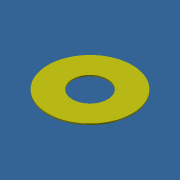
# Autodesk Inventor part: plancha
Saved by Autodesk Inventor 2014 (Build 180170000, 170)
## iProperties
Created: 2014-03-15
Part Number: plancha
Material: Generic
Document SubType Name: Modeling
Designer: Lefo
Density: 1 g/cm^3
Appearance: Default
Author: Lefo
Autodesk Inventor part; units mm, degrees
ref_plane "YZ Plane" through (0, 0, 0) normal (1, 0, 0) x (0, 1, 0)
ref_plane "XZ Plane" through (0, 0, 0) normal (0, 1, 0) x (-1, 0, 0)
ref_plane "XY Plane" through (0, 0, 0) normal (0, 0, 1) x (1, 0, 0)
sketch "Sketch1" plane through (0, 0, 0) normal (0, 1, 0) x (-1, 0, 0)
  line L0 (1200, -600) -> (-1200, -600)
  line L1 (-1200, -600) -> (-1200, 600)
  line L2 (-1200, 600) -> (1200, 600)
  line L3 (1200, 600) -> (1200, -600)
  line L4 (1200, -600) -> (-1200, 600) construction
  line L5 (-1200, -600) -> (1200, 600) construction
  circle A0 centre (0, 0) radius 130 construction
  circle A1 centre (0, 0) radius 325 construction
  line L6 (0, 325) -> (309.0934, 100.4305) construction
  line L7 (309.0934, 100.4305) -> (191.0302, -262.9305) construction
  line L8 (191.0302, -262.9305) -> (-191.0302, -262.9305) construction
  line L9 (-191.0302, -262.9305) -> (-309.0934, 100.4305) construction
  line L10 (-309.0934, 100.4305) -> (0, 325) construction
  line L11 (0, 0) -> (0, 325) construction
  line L12 (0, 0) -> (-309.0934, 100.4305) construction
  line L13 (0, 0) -> (-191.0302, -262.9305) construction
  line L14 (0, 0) -> (309.0934, 100.4305) construction
  line L15 (0, 0) -> (191.0302, -262.9305) construction
  arc A2 (-15.7737, 293.9464) -> (0, 0) centre (281.4583, 162.5) ccw
  arc A3 (224.7845, 110.9324) -> (0, 0) centre (230.7976, -184.461) ccw
  arc A4 (275.3692, 201.188) -> (35.5667, 329.5753) centre (50.8772, 70.0265) ccw
  arc A5 (224.7845, 110.9324) -> (275.3692, 201.188) centre (223.5633, 170.92) ccw
  arc A6 (35.5667, 329.5753) -> (-15.7737, 293.9464) centre (39.0999, 269.6794) ccw
  arc A7 (-284.434, 75.8328) -> (0, 0) centre (-67.5713, 317.898) ccw
  arc A8 (-36.0407, 248.0627) -> (0, 0) centre (246.7532, 162.5) ccw
  arc A9 (-106.2474, 324.0622) -> (-302.454, 135.6703) centre (-50.8772, 70.0265) ccw
  arc A10 (-36.0407, 248.0627) -> (-106.2474, 324.0622) centre (-93.4697, 265.4385) ccw
  arc A11 (-302.454, 135.6703) -> (-284.434, 75.8328) centre (-244.3978, 120.5217) ccw
  arc A12 (-160.0162, -247.0792) -> (0, 0) centre (-323.2196, 33.9718) ccw
  arc A13 (-247.0589, 42.3788) -> (0, 0) centre (-78.2958, 284.8915) ccw
  arc A14 (-341.0337, -0.9066) -> (-222.4935, -245.7264) centre (-82.321, -26.7477) ccw
  arc A15 (-247.0589, 42.3788) -> (-341.0337, -0.9066) centre (-281.3308, -6.8699) ccw
  arc A16 (-222.4935, -245.7264) -> (-160.0162, -247.0792) centre (-190.146, -195.1929) ccw
  arc A17 (185.5386, -228.5361) -> (0, 0) centre (-132.1894, -296.9023) ccw
  arc A18 (-116.65, -221.8712) -> (0, 0) centre (-295.1426, 13.5726) ccw
  arc A19 (-104.523, -324.6224) -> (164.9454, -287.5376) centre (0, -86.5575) ccw
  arc A20 (-116.65, -221.8712) -> (-104.523, -324.6224) centre (-80.4023, -269.6844) ccw
  arc A21 (164.9454, -287.5376) -> (185.5386, -228.5361) centre (126.8811, -241.1575) ccw
  arc A22 (274.6853, 105.8361) -> (0, 0) centre (241.5221, -217.4674) ccw
  arc A23 (174.9652, -179.5027) -> (0, 0) centre (-104.1124, -276.5031) ccw
  arc A24 (276.4349, -199.7211) -> (324.4354, 68.0184) centre (82.321, -26.7477) ccw
  arc A25 (174.9652, -179.5027) -> (276.4349, -199.7211) centre (231.6394, -159.8042) ccw
  arc A26 (324.4354, 68.0184) -> (274.6853, 105.8361) centre (268.5629, 46.1493) ccw
  line L16 (246.7532, 162.5) -> (-78.2958, 284.8915)
  line L17 (-78.2958, 284.8915) -> (-295.1426, 13.5726)
  line L18 (-295.1426, 13.5726) -> (-104.1124, -276.5031)
  line L19 (-104.1124, -276.5031) -> (230.7976, -184.461)
  line L20 (230.7976, -184.461) -> (246.7532, 162.5)
  circle A27 centre (0, 0) radius 251.1364
  circle A28 centre (223.5633, 170.92) radius 60 construction
  circle A29 centre (246.7532, 162.5) radius 43.2425 construction
  circle A30 centre (246.7532, 162.5) radius 3.5
  circle A31 centre (39.0999, 269.6794) radius 3.5
  circle A32 centre (-78.2958, 284.8915) radius 3.5
  circle A33 centre (-244.3978, 120.5217) radius 3.5
  circle A34 centre (-295.1426, 13.5726) radius 3.5
  circle A35 centre (-190.146, -195.1929) radius 3.5
  circle A36 centre (-104.1124, -276.5031) radius 3.5
  circle A37 centre (126.8811, -241.1575) radius 3.5
  circle A38 centre (230.7976, -184.461) radius 3.5
  circle A39 centre (268.5629, 46.1493) radius 3.5
  point P0 (-309.0934, 100.4305)
  point P1 (0, 325)
  point P2 (-191.0302, -262.9305)
  point P3 (-309.0934, 100.4305)
  point P4 (191.0302, -262.9305)
  point P5 (-191.0302, -262.9305)
  point P6 (309.0934, 100.4305)
  point P7 (191.0302, -262.9305)
  dimension "d3" = 650
  dimension "d0" = 2400
  dimension "d1" = 1200
  dimension "d2" = 260
  dimension "d9" = 325
  dimension "d10" = 295.4545
  dimension "d11" = 260
  dimension "d12" = 60
  dimension "d15" = 360
  dimension "d21" = 502.2727
  dimension "d22" = 7
  dimension "d23" = 7
  dimension "d24" = 7
  dimension "d25" = 7
  dimension "d26" = 7
  dimension "d27" = 7
  dimension "d28" = 7
  dimension "d29" = 7
  dimension "d30" = 7
  dimension "d31" = 7
  constraints: 70 point on circle, 42 end point, 39 centre point, 15 coincident, 6 perpendicular, 4 tangent, 2 equal radius, 2 parallel, 1 horizontal, 1 vertical alignment, 99 other
  measures "d0" distance of L1.end L2.end
  measures "d1" distance of L0.end L1.end
  measures "d2" diameter of A0
  measures "d9" radius of A2
  measures "d10" radius of A3
  measures "d11" radius of A4
  measures "d12" radius of A5
  measures "d21" diameter of A27
  measures "d22" diameter of A30
  measures "d23" diameter of A31
  measures "d24" diameter of A32
  measures "d25" diameter of A33
  measures "d26" diameter of A34
  measures "d27" diameter of A35
  measures "d28" diameter of A36
  measures "d29" diameter of A37
  measures "d30" diameter of A38
  measures "d31" diameter of A39
extrude "Extrusion1" add sketch "Sketch1" along normal blind 19 contours L0 L1 L2 L3 | A6 A4 A5 L20 A30 L16 A27 A2 | L16 A27 A2 | A2 A27 A10 L16 | A27 L16 A5 A3 A2 | A2 A8 A10 A27 | A27 L16 | L16 A32 L17 A27 A7 A11 A9 A10 | A10 A27 L17 A32 L16 | A13 A15 A27 A7 | A7 A27 L17 A10 A8 | A18 A20 A27 A12 | A12 A27 L18 A15 A13 | A23 A25 A27 A17 | A17 A27 L19 A20 A18 | A3 A5 A27 A22 | A22 A27 L20 A25 A23 | L16 A30 L20 A5 A27 | A32 L17 L16 | L16 L17 A32 | L20 A22 A27 A5 | A27 A15 L17 A7 | A7 L17 A27 | A27 A20 L18 A12 | A12 L18 A27 | A27 A25 L19 A17 | A17 L19 A27 | A22 L20 A27 | L17 A27 | A30 L20 L16 | L16 L20 A30 | A22 A26 A24 A25 L19 A38 L20 A27 | A27 L18 A34 L17 A15 | A12 A16 A14 A15 L17 A34 L18 A27 | A27 L18 | A27 L19 A36 L18 A20 | A17 A21 A19 A20 L18 A36 L19 A27 | A27 L19 | A27 L20 A38 L19 A25 | A27 L20 | A34 L18 L17 | L17 L18 A34 | A36 L19 L18 | L18 L19 A36 | A38 L20 L19 | L19 L20 A38 | A31 | A33 | A35 | A37 | A39
extrude "Extrusion3" cut sketch "Sketch1" along normal blind 19 contours A32 L17 L16 | L16 L17 A32 | A30 L20 L16 | L16 L20 A30 | A34 L18 L17 | L17 L18 A34 | A36 L19 L18 | L18 L19 A36 | A38 L20 L19 | L19 L20 A38 | A31 | A33 | A35 | A37 | A39
sketch "Sketch3" plane through (0, 0, 0) normal (0, -1, 0) x (1, 0, 0)
  circle A0 centre (0, 0) radius 251.1364 projected
extrude "Extrusion4" cut sketch "Sketch3" against normal up to next
sketch "Sketch7" plane through (0, 0, 0) normal (0, -1, 0) x (1, 0, 0)
  arc A0 (-0.1434, 553) -> (-0.1452, 560) centre (-0.1443, 556.5) ccw projected
  circle A1 centre (-0.1443, 556.5) radius 3.18
  dimension "d50" = 6.36
  constraints: 1 centre point, 1 coincident
  measures "d50" diameter of A1
extrude "Extrusion8" cut sketch "Sketch7" against normal blind 19
pattern_circular "Circular Pattern1" count 5 over 360 about axis through (0, 0, 0) along (0, 1, 0) of "Extrusion8"
sketch "Sketch8" plane through (0, 0, 0) normal (0, -1, 0) x (1, 0, 0)
  circle A0 centre (0, 0) radius 251.1364 projected
  line L0 (-1200, -600) -> (1200, -600) projected
  line L1 (1200, -600) -> (1200, 600) projected
  line L2 (1200, 600) -> (-1200, 600) projected
  line L3 (-1200, 600) -> (-1200, -600) projected
  circle A1 centre (0, 0) radius 600
  dimension "d47" = 1200
  constraints: 1 centre point, 1 coincident
  measures "d47" diameter of A1
extrude "Extrusion9" cut sketch "Sketch8" against normal blind 19 contours A0 | L3 L2 A1 L0 | A1 L2 L1 L0
equation "\"d2\" = 0.4 * d3"
equation "\"d9\" = 0.5 * d3"
equation "\"d10\" = 0.454545 * d3"
equation "\"d11\" = 0.4 * d3"
equation "\"d21\" = 1.7 * d10"
body "Solid1"
